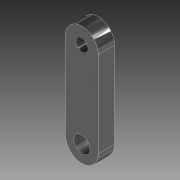
# Autodesk Inventor part: Dog Shifter Reverse Connector Plate
Saved by Autodesk Inventor 2021 (Build 250183000, 183)
## iProperties
Created: 2021-04-11
Part Number: Dog Shifter Reverse Connector Plate
Material: Aluminum 6061
Document SubType Name: Modeling
Designer: Cal
Density: 2.7 g/cm^3
Appearance: Glazed - Black
Author: Cal
Autodesk Inventor part; units mm, degrees
ref_plane "YZ Plane" through (0, 0, 0) normal (1, 0, 0) x (0, 1, 0)
ref_plane "XZ Plane" through (0, 0, 0) normal (0, 1, 0) x (-1, 0, 0)
ref_plane "XY Plane" through (0, 0, 0) normal (0, 0, 1) x (1, 0, 0)
sketch "Sketch1" plane through (0, 0, 0) normal (0, 0, 1) x (1, 0, 0)
  line L0 (0, -16.6688) -> (0, 16.6688) construction
  line L1 (-6.35, -16.6688) -> (-6.35, 16.6688)
  line L2 (6.35, 16.6688) -> (6.35, -16.6687)
  arc A0 (-6.35, -16.6688) -> (6.35, -16.6687) centre (0, -16.6688) ccw
  arc A1 (6.35, 16.6688) -> (-6.35, 16.6688) centre (0, 16.6688) ccw
  circle A2 centre (0, 16.6688) radius 2.413
  circle A3 centre (0, -16.6688) radius 3.175
  point P0 (0, 0)
  dimension "d0" = 16.6687
  dimension "d1" = 4.826
  dimension "d2" = 6.35
  dimension "d3" = 6.35
  constraints: 8 end point, 4 centre point, 4 point on circle, 4 tangent, 2 coincident, 1 midpoint, 1 parallel, 1 vertical
  measures "d0" distance of point (0, 0) L0.end
  measures "d1" diameter of A2
  measures "d2" diameter of A3
  measures "d3" radius of A0
extrude "Extrusion1" add sketch "Sketch1" along normal blind 6.35
body "Solid1"
